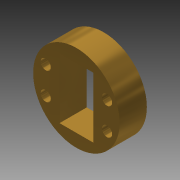
# Autodesk Inventor part: WG18FLANGECutDown
Saved by Autodesk Inventor 2015 (Build 190159000, 159)
## iProperties
Created: 2014-03-25
Part Number: WG18FLANGECutDown
Material: Brass, Soft Yellow
Document SubType Name: Modeling
Designer: jad211
Density: 8.47 g/cm^3
Appearance: Brass - Satin
Author: jad211
Autodesk Inventor part; units mm, degrees
ref_plane "YZ Plane" through (0, 0, 0) normal (1, 0, 0) x (0, 1, 0)
ref_plane "XZ Plane" through (0, 0, 0) normal (0, 1, 0) x (-1, 0, 0)
ref_plane "XY Plane" through (0, 0, 0) normal (0, 0, 1) x (1, 0, 0)
sketch "Sketch3" plane through (0, 0, 0) normal (0, 0, 1) x (1, 0, 0)
  line L0 (-15.8918, -16.7) -> (15.8918, -16.7)
  line L1 (16.7, -15.7) -> (16.7, 15.7)
  line L2 (15.8918, 16.7) -> (-15.8918, 16.7)
  line L3 (-16.7, 15.7) -> (-16.7, -15.7)
  line L4 (-15.8918, 16.7) -> (-16.7, 15.7)
  line L5 (15.8918, 16.7) -> (16.7, 15.7)
  line L6 (16.7, -15.7) -> (15.8918, -16.7)
  line L7 (-16.7, -15.7) -> (-15.8918, -16.7)
  line L8 (-4.9497, -8.8994) -> (4.9497, -8.8994)
  line L9 (4.9497, -8.8994) -> (4.9497, 8.8994)
  line L10 (4.9497, 8.8994) -> (-4.9497, 8.8994)
  line L11 (-4.9497, 8.8994) -> (-4.9497, -8.8994)
  circle A0 centre (-12.14, 12.625) radius 2.045
  circle A1 centre (12.14, 12.625) radius 2.045
  line L12 (0, -16.7) -> (0, 16.7) construction
  circle A2 centre (-12.14, -12.625) radius 2.045
  circle A3 centre (12.14, -12.625) radius 2.045
  line L13 (12.14, 12.625) -> (-12.14, 12.625) construction
  line L14 (-12.14, 12.625) -> (-12.14, -12.625) construction
  line L15 (-12.14, -12.625) -> (12.14, -12.625) construction
  line L16 (12.14, -12.625) -> (12.14, 12.625) construction
  line L17 (-16.7, 0) -> (16.7, 0) construction
  circle A4 centre (0, 0) radius 18.4 construction
  circle A5 centre (-9, 4) radius 1.5
  circle A6 centre (9, 4) radius 1.5
  circle A7 centre (-9, -4) radius 1.5
  circle A8 centre (9, -4) radius 1.5
  dimension "d10" = 9.8994
  dimension "d11" = 17.7988
  dimension "d12" = 4.09
  dimension "d13" = 4.09
  dimension "d17" = 4.09
  dimension "d19" = 24.28
  dimension "d20" = 25.25
  dimension "d21" = 4.09
  dimension "d22" = 12.625
  dimension "d26" = 36.8
  dimension "d38" = 12.14
  dimension "d39" = 33.4
  dimension "d40" = 33.4
  dimension "d45" = 3
  dimension "d46" = 3
  dimension "d47" = 3
  dimension "d48" = 3
  dimension "d49" = 4
  dimension "d57" = 8.8994
  dimension "d58" = 4.9497
  dimension "d59" = 9
  dimension "d60" = 9
  dimension "d61" = 9
  dimension "d62" = 9
  dimension "d63" = 4
  dimension "d64" = 4
  dimension "d65" = 4
  constraints: 37 end point, 9 centre point, 6 midpoint, 6 perpendicular, 4 parallel, 2 coincident, 2 horizontal
  measures "d10" distance of L10.end L9.end
  measures "d11" distance of L9.end L8.end
  measures "d12" diameter of A0
  measures "d13" diameter of A1
  measures "d17" diameter of A2
  measures "d19" distance of L13.start L13.end
  measures "d20" distance of L14.end L13.end
  measures "d21" diameter of A3
  measures "d22" distance from line of L17.start L13
  measures "d26" diameter of A4
  measures "d38" distance from line of L12 L13.end
  measures "d39" distance of L0.end L2.start
  measures "d40" distance of L3.end L1.start
  measures "d45" diameter of A5
  measures "d46" diameter of A6
  measures "d47" diameter of A7
  measures "d48" diameter of A8
  measures "d49" distance from line of A5.centre L17
  measures "d57" distance from line of L8 point (0, 0)
  measures "d58" horizontal distance of point (0, 0) L9.end
  measures "d59" distance from line of L12 A5.centre
  measures "d60" distance from line of L12 A7.centre
  measures "d61" distance from line of L12 A6.centre
  measures "d62" distance from line of L12 A8.centre
  measures "d63" distance from line of L17 A7.centre
  measures "d64" distance from line of L17 A8.centre
  measures "d65" distance from line of L17 A6.centre
sketch "Sketch4" plane through (0, 0, 0) normal (0, 0, 1) x (1, 0, 0)
  circle A0 centre (0, 0) radius 12.7
  dimension "d32" = 25.4
  constraints: 1 centre point, 1 coincident
  measures "d32" diameter of A0
extrude "Extrusion5" add sketch "Sketch3" along normal blind 8
extrude "Extrusion6" cut sketch "Sketch4" along normal blind 8 keep common part
body "Solid3"
